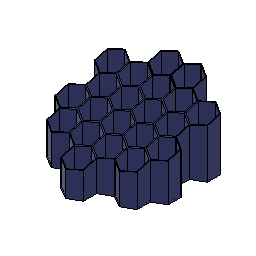
hexagon-06 (Autodesk Fusion 360 design; units mm, degrees)
Autodesk Fusion 360 part; units mm, degrees
sketch "Sketch1" plane through (0, 0, 0) normal (0, 1, 0) x (1, 0, 0)
  line L0 (15.0321, 8.6045) -> (0.0644, 17.3204)
  line L1 (0.0644, 17.3204) -> (-14.9677, 8.7159)
  line L2 (-14.9677, 8.7159) -> (-15.0321, -8.6045)
  line L3 (-15.0321, -8.6045) -> (-0.0644, -17.3204)
  line L4 (-0.0644, -17.3204) -> (14.9677, -8.7159)
  line L5 (14.9677, -8.7159) -> (15.0321, 8.6045)
  line L6 (14.9677, -8.7159) -> (-0.0644, -17.3204)
  line L7 (-0.0644, -17.3204) -> (-0.1287, -34.6408)
  line L8 (-0.1287, -34.6408) -> (14.839, -43.3567)
  line L9 (14.839, -43.3567) -> (29.8711, -34.7523)
  line L10 (29.8711, -34.7523) -> (29.9354, -17.4319)
  line L11 (29.9354, -17.4319) -> (14.9677, -8.7159)
  line L12 (14.839, -43.3567) -> (-0.1287, -34.6408)
  line L13 (-0.1287, -34.6408) -> (-15.1608, -43.2452)
  line L14 (-15.1608, -43.2452) -> (-15.2252, -60.5656)
  line L15 (-15.2252, -60.5656) -> (-0.2575, -69.2816)
  line L16 (-0.2575, -69.2816) -> (14.7746, -60.6771)
  line L17 (14.7746, -60.6771) -> (14.839, -43.3567)
  line L18 (14.2, 8.1984) -> (0, 16.3967)
  line L19 (0, 16.3967) -> (-14.2, 8.1984)
  line L20 (-14.2, 8.1984) -> (-14.2, -8.1984)
  line L21 (-14.2, -8.1984) -> (0, -16.3967)
  line L22 (0, -16.3967) -> (14.2, -8.1984)
  line L23 (14.2, -8.1984) -> (14.2, 8.1984)
  line L24 (29.1033, -17.838) -> (14.9033, -9.6396)
  line L25 (14.9033, -9.6396) -> (0.7033, -17.838)
  line L26 (0.7033, -17.838) -> (0.7033, -34.2347)
  line L27 (0.7033, -34.2347) -> (14.9033, -42.4331)
  line L28 (14.9033, -42.4331) -> (29.1033, -34.2347)
  line L29 (29.1033, -34.2347) -> (29.1033, -17.838)
  line L30 (14.0069, -43.7628) -> (-0.1931, -35.5644)
  line L31 (-0.1931, -35.5644) -> (-14.3931, -43.7628)
  line L32 (-14.3931, -43.7628) -> (-14.3931, -60.1595)
  line L33 (-14.3931, -60.1595) -> (-0.1931, -68.3579)
  line L34 (-0.1931, -68.3579) -> (14.0069, -60.1595)
  line L35 (14.0069, -60.1595) -> (14.0069, -43.7628)
  line L36 (14.7746, -60.6771) -> (-0.2575, -69.2816)
  line L37 (-0.2575, -69.2816) -> (-0.3218, -86.6019)
  line L38 (-0.3218, -86.6019) -> (14.6459, -95.3179)
  line L39 (14.6459, -95.3179) -> (29.678, -86.7134)
  line L40 (29.678, -86.7134) -> (29.7423, -69.393)
  line L41 (29.7423, -69.393) -> (14.7746, -60.6771)
  line L42 (28.9103, -69.7991) -> (14.7103, -61.6007)
  line L43 (14.7103, -61.6007) -> (0.5103, -69.7991)
  line L44 (0.5103, -69.7991) -> (0.5103, -86.1959)
  line L45 (0.5103, -86.1959) -> (14.7103, -94.3942)
  line L46 (14.7103, -94.3942) -> (28.9103, -86.1959)
  line L47 (28.9103, -86.1959) -> (28.9103, -69.7991)
  line L48 (44.7746, -60.6771) -> (29.7425, -69.2816)
  line L49 (44.9677, -8.7159) -> (45.0321, 8.6045)
  line L50 (44.9033, -9.6396) -> (30.7033, -17.838)
  line L51 (29.9356, -17.3204) -> (44.9677, -8.7159)
  line L52 (15.8, 8.1984) -> (15.8, -8.1984)
  line L53 (14.7748, -60.5656) -> (29.7425, -69.2816)
  line L54 (30, -16.3967) -> (44.2, -8.1984)
  line L55 (29.7425, -69.2816) -> (29.6782, -86.6019)
  line L56 (44.7103, -61.6007) -> (30.5103, -69.7991)
  line L57 (29.8069, -68.3579) -> (44.0069, -60.1595)
  line L58 (45.0321, 8.6045) -> (30.0644, 17.3204)
  line L59 (15.0323, 8.7159) -> (14.9679, -8.6045)
  line L60 (30.5103, -69.7991) -> (30.5103, -86.1959)
  line L61 (30.7033, -17.838) -> (30.7033, -34.2347)
  line L62 (29.8713, -34.6408) -> (14.8392, -43.2452)
  line L63 (15.8, -8.1984) -> (30, -16.3967)
  line L64 (30, 16.3967) -> (15.8, 8.1984)
  line L65 (29.8069, -35.5644) -> (15.6069, -43.7628)
  line L66 (44.839, -43.3567) -> (29.8713, -34.6408)
  line L67 (30.0644, 17.3204) -> (15.0323, 8.7159)
  line L68 (44.0069, -43.7628) -> (29.8069, -35.5644)
  line L69 (29.9356, -17.3204) -> (29.8713, -34.6408)
  line L70 (44.2, -8.1984) -> (44.2, 8.1984)
  line L71 (30.7033, -34.2347) -> (44.9033, -42.4331)
  line L72 (44.9677, -8.7159) -> (29.9356, -17.3204)
  line L73 (44.2, 8.1984) -> (30, 16.3967)
  line L74 (58.9103, -69.7991) -> (44.7103, -61.6007)
  line L75 (59.9354, -17.4319) -> (44.9677, -8.7159)
  line L76 (59.7423, -69.393) -> (44.7746, -60.6771)
  line L77 (44.9033, -42.4331) -> (59.1033, -34.2347)
  line L78 (59.678, -86.7134) -> (59.7423, -69.393)
  line L79 (59.1033, -17.838) -> (44.9033, -9.6396)
  line L80 (44.6459, -95.3179) -> (59.678, -86.7134)
  line L81 (44.839, -43.3567) -> (59.8711, -34.7523)
  line L82 (59.8711, -34.7523) -> (59.9354, -17.4319)
  line L83 (59.1033, -34.2347) -> (59.1033, -17.838)
  line L84 (15.6069, -60.1595) -> (29.8069, -68.3579)
  line L85 (44.0069, -60.1595) -> (44.0069, -43.7628)
  line L86 (29.6782, -86.6019) -> (44.6459, -95.3179)
  line L87 (30.5103, -86.1959) -> (44.7103, -94.3942)
  line L88 (14.9679, -8.6045) -> (29.9356, -17.3204)
  line L89 (29.7425, -69.2816) -> (44.7746, -60.6771)
  line L90 (29.8713, -34.6408) -> (44.839, -43.3567)
  line L91 (58.9103, -86.1959) -> (58.9103, -69.7991)
  line L92 (44.7103, -94.3942) -> (58.9103, -86.1959)
  line L93 (44.7746, -60.6771) -> (44.839, -43.3567)
  line L94 (14.8392, -43.2452) -> (14.7748, -60.5656)
  line L95 (15.6069, -43.7628) -> (15.6069, -60.1595)
  line L96 (74.7746, -60.6771) -> (59.7425, -69.2816)
  line L97 (74.9677, -8.7159) -> (75.0321, 8.6045)
  line L98 (74.9033, -9.6396) -> (60.7033, -17.838)
  line L99 (59.9356, -17.3204) -> (74.9677, -8.7159)
  line L100 (45.8, 8.1984) -> (45.8, -8.1984)
  line L101 (44.7748, -60.5656) -> (59.7425, -69.2816)
  line L102 (60, -16.3967) -> (74.2, -8.1984)
  line L103 (59.7425, -69.2816) -> (59.6782, -86.6019)
  line L104 (74.7103, -61.6007) -> (60.5103, -69.7991)
  line L105 (59.8069, -68.3579) -> (74.0069, -60.1595)
  line L106 (75.0321, 8.6045) -> (60.0644, 17.3204)
  line L107 (45.0323, 8.7159) -> (44.9679, -8.6045)
  line L108 (60.5103, -69.7991) -> (60.5103, -86.1959)
  line L109 (60.7033, -17.838) -> (60.7033, -34.2347)
  line L110 (59.8713, -34.6408) -> (44.8392, -43.2452)
  line L111 (45.8, -8.1984) -> (60, -16.3967)
  line L112 (60, 16.3967) -> (45.8, 8.1984)
  line L113 (59.8069, -35.5644) -> (45.6069, -43.7628)
  line L114 (74.839, -43.3567) -> (59.8713, -34.6408)
  line L115 (60.0644, 17.3204) -> (45.0323, 8.7159)
  line L116 (74.0069, -43.7628) -> (59.8069, -35.5644)
  line L117 (59.9356, -17.3204) -> (59.8713, -34.6408)
  line L118 (74.2, -8.1984) -> (74.2, 8.1984)
  line L119 (60.7033, -34.2347) -> (74.9033, -42.4331)
  line L120 (74.9677, -8.7159) -> (59.9356, -17.3204)
  line L121 (74.2, 8.1984) -> (60, 16.3967)
  line L122 (88.9103, -69.7991) -> (74.7103, -61.6007)
  line L123 (89.9354, -17.4319) -> (74.9677, -8.7159)
  line L124 (89.7423, -69.393) -> (74.7746, -60.6771)
  line L125 (74.9033, -42.4331) -> (89.1033, -34.2347)
  line L126 (89.678, -86.7134) -> (89.7423, -69.393)
  line L127 (89.1033, -17.838) -> (74.9033, -9.6396)
  line L128 (74.6459, -95.3179) -> (89.678, -86.7134)
  line L129 (74.839, -43.3567) -> (89.8711, -34.7523)
  line L130 (89.8711, -34.7523) -> (89.9354, -17.4319)
  line L131 (89.1033, -34.2347) -> (89.1033, -17.838)
  line L132 (45.6069, -60.1595) -> (59.8069, -68.3579)
  line L133 (74.0069, -60.1595) -> (74.0069, -43.7628)
  line L134 (59.6782, -86.6019) -> (74.6459, -95.3179)
  line L135 (60.5103, -86.1959) -> (74.7103, -94.3942)
  line L136 (44.9679, -8.6045) -> (59.9356, -17.3204)
  line L137 (59.7425, -69.2816) -> (74.7746, -60.6771)
  line L138 (59.8713, -34.6408) -> (74.839, -43.3567)
  line L139 (88.9103, -86.1959) -> (88.9103, -69.7991)
  line L140 (74.7103, -94.3942) -> (88.9103, -86.1959)
  line L141 (74.7746, -60.6771) -> (74.839, -43.3567)
  line L142 (44.8392, -43.2452) -> (44.7748, -60.5656)
  line L143 (45.6069, -43.7628) -> (45.6069, -60.1595)
  line L144 (104.7746, -60.6771) -> (89.7425, -69.2816)
  line L145 (104.9677, -8.7159) -> (105.0321, 8.6045)
  line L146 (104.9033, -9.6396) -> (90.7033, -17.838)
  line L147 (89.9356, -17.3204) -> (104.9677, -8.7159)
  line L148 (75.8, 8.1984) -> (75.8, -8.1984)
  line L149 (74.7748, -60.5656) -> (89.7425, -69.2816)
  line L150 (90, -16.3967) -> (104.2, -8.1984)
  line L151 (89.7425, -69.2816) -> (89.6782, -86.6019)
  line L152 (104.7103, -61.6007) -> (90.5103, -69.7991)
  line L153 (89.8069, -68.3579) -> (104.0069, -60.1595)
  line L154 (105.0321, 8.6045) -> (90.0644, 17.3204)
  line L155 (75.0323, 8.7159) -> (74.9679, -8.6045)
  line L156 (90.5103, -69.7991) -> (90.5103, -86.1959)
  line L157 (90.7033, -17.838) -> (90.7033, -34.2347)
  line L158 (89.8713, -34.6408) -> (74.8392, -43.2452)
  line L159 (75.8, -8.1984) -> (90, -16.3967)
  line L160 (90, 16.3967) -> (75.8, 8.1984)
  line L161 (89.8069, -35.5644) -> (75.6069, -43.7628)
  line L162 (104.839, -43.3567) -> (89.8713, -34.6408)
  line L163 (90.0644, 17.3204) -> (75.0323, 8.7159)
  line L164 (104.0069, -43.7628) -> (89.8069, -35.5644)
  line L165 (89.9356, -17.3204) -> (89.8713, -34.6408)
  line L166 (104.2, -8.1984) -> (104.2, 8.1984)
  line L167 (90.7033, -34.2347) -> (104.9033, -42.4331)
  line L168 (104.9677, -8.7159) -> (89.9356, -17.3204)
  line L169 (104.2, 8.1984) -> (90, 16.3967)
  line L170 (118.9103, -69.7991) -> (104.7103, -61.6007)
  line L171 (119.9354, -17.4319) -> (104.9677, -8.7159)
  line L172 (119.7423, -69.393) -> (104.7746, -60.6771)
  line L173 (104.9033, -42.4331) -> (119.1033, -34.2347)
  line L174 (119.678, -86.7134) -> (119.7423, -69.393)
  line L175 (119.1033, -17.838) -> (104.9033, -9.6396)
  line L176 (104.6459, -95.3179) -> (119.678, -86.7134)
  line L177 (104.839, -43.3567) -> (119.8711, -34.7523)
  line L178 (119.8711, -34.7523) -> (119.9354, -17.4319)
  line L179 (119.1033, -34.2347) -> (119.1033, -17.838)
  line L180 (75.6069, -60.1595) -> (89.8069, -68.3579)
  line L181 (104.0069, -60.1595) -> (104.0069, -43.7628)
  line L182 (89.6782, -86.6019) -> (104.6459, -95.3179)
  line L183 (90.5103, -86.1959) -> (104.7103, -94.3942)
  line L184 (74.9679, -8.6045) -> (89.9356, -17.3204)
  line L185 (89.7425, -69.2816) -> (104.7746, -60.6771)
  line L186 (89.8713, -34.6408) -> (104.839, -43.3567)
  line L187 (118.9103, -86.1959) -> (118.9103, -69.7991)
  line L188 (104.7103, -94.3942) -> (118.9103, -86.1959)
  line L189 (104.7746, -60.6771) -> (104.839, -43.3567)
  line L190 (74.8392, -43.2452) -> (74.7748, -60.5656)
  line L191 (75.6069, -43.7628) -> (75.6069, -60.1595)
  line L192 (30.0644, 17.3204) -> (45.0323, 8.7159)
  line L193 (45.0323, 8.7159) -> (59.9679, 17.3763)
  line L194 (59.9679, 17.3763) -> (59.9356, 34.6411)
  line L195 (59.9356, 34.6411) -> (44.9677, 43.2456)
  line L196 (44.9677, 43.2456) -> (30.0321, 34.5852)
  line L197 (30.0321, 34.5852) -> (30.0644, 17.3204)
  line L198 (59.9679, 17.3763) -> (75.0323, 8.7159)
  line L199 (75.0323, 8.7159) -> (90.0646, 17.4319)
  line L200 (90.0646, 17.4319) -> (90.0325, 34.8082)
  line L201 (90.0325, 34.8082) -> (74.9681, 43.4686)
  line L202 (74.9681, 43.4686) -> (59.9358, 34.7526)
  line L203 (59.9358, 34.7526) -> (59.9679, 17.3763)
  line L204 (104.9677, -8.7159) -> (119.9354, -17.4319)
  line L205 (119.9354, -17.4319) -> (134.9675, -8.8274)
  line L206 (134.9675, -8.8274) -> (135.0319, 8.493)
  line L207 (135.0319, 8.493) -> (120.0642, 17.2089)
  line L208 (120.0642, 17.2089) -> (105.0321, 8.6045)
  line L209 (105.0321, 8.6045) -> (104.9677, -8.7159)
  line L210 (104.839, -43.3567) -> (104.7746, -60.6771)
  line L211 (104.7746, -60.6771) -> (119.7423, -69.393)
  line L212 (119.7423, -69.393) -> (134.7744, -60.7886)
  line L213 (134.7744, -60.7886) -> (134.8388, -43.4682)
  line L214 (134.8388, -43.4682) -> (119.8711, -34.7523)
  line L215 (119.8711, -34.7523) -> (104.839, -43.3567)
  line L216 (44.6459, -95.3179) -> (44.678, -112.6942)
  line L217 (44.678, -112.6942) -> (59.7423, -121.3546)
  line L218 (59.7423, -121.3546) -> (74.7746, -112.6386)
  line L219 (74.7746, -112.6386) -> (74.7425, -95.2623)
  line L220 (74.7425, -95.2623) -> (59.6782, -86.6019)
  line L221 (59.6782, -86.6019) -> (44.6459, -95.3179)
  line L222 (59.2161, 34.1512) -> (45.0323, 42.3775)
  line L223 (45.0323, 42.3775) -> (30.8162, 34.2071)
  line L224 (30.8162, 34.2071) -> (30.7839, 17.8104)
  line L225 (30.7839, 17.8104) -> (44.9677, 9.584)
  line L226 (44.9677, 9.584) -> (59.1838, 17.7544)
  line L227 (59.1838, 17.7544) -> (59.2161, 34.1512)
  line L228 (89.2002, 34.2906) -> (75.0002, 42.489)
  line L229 (75.0002, 42.489) -> (60.8002, 34.2906)
  line L230 (60.8002, 34.2906) -> (60.8002, 17.8939)
  line L231 (60.8002, 17.8939) -> (75.0002, 9.6955)
  line L232 (75.0002, 9.6955) -> (89.2002, 17.8939)
  line L233 (89.2002, 17.8939) -> (89.2002, 34.2906)
  line L234 (134.0371, -43.9271) -> (119.8676, -35.676)
  line L235 (119.8676, -35.676) -> (105.6373, -43.8216)
  line L236 (105.6373, -43.8216) -> (105.5763, -60.2182)
  line L237 (105.5763, -60.2182) -> (119.7458, -68.4693)
  line L238 (119.7458, -68.4693) -> (133.9761, -60.3237)
  line L239 (133.9761, -60.3237) -> (134.0371, -43.9271)
  line L240 (134.2302, 8.0341) -> (120.0607, 16.2852)
  line L241 (120.0607, 16.2852) -> (105.8304, 8.1396)
  line L242 (105.8304, 8.1396) -> (105.7694, -8.257)
  line L243 (105.7694, -8.257) -> (119.9389, -16.5081)
  line L244 (119.9389, -16.5081) -> (134.1692, -8.3626)
  line L245 (134.1692, -8.3626) -> (134.2302, 8.0341)
  line L246 (73.8951, -95.7537) -> (59.68, -87.5815)
  line L247 (59.68, -87.5815) -> (45.4951, -95.8061)
  line L248 (45.4951, -95.8061) -> (45.5254, -112.2028)
  line L249 (45.5254, -112.2028) -> (59.7405, -120.375)
  line L250 (59.7405, -120.375) -> (73.9254, -112.1504)
  line L251 (73.9254, -112.1504) -> (73.8951, -95.7537)
  point P0 (14.9033, -26.0363)
  point P1 (-0.1931, -51.9612)
  point P2 (14.9033, -26.0363)
  point P3 (-0.1931, -51.9612)
  point P4 (14.7103, -77.9975)
  point P5 (14.7103, -77.9975)
  point P6 (44.9033, -26.0363)
  point P7 (29.8069, -51.9612)
  point P8 (44.9033, -26.0363)
  point P9 (30, 0)
  point P10 (30, 0)
  point P11 (29.8069, -51.9612)
  point P12 (44.7103, -77.9975)
  point P13 (30, 0)
  point P14 (44.7103, -77.9975)
  point P15 (74.9033, -26.0363)
  point P16 (59.8069, -51.9612)
  point P17 (74.9033, -26.0363)
  point P18 (60, 0)
  point P19 (60, 0)
  point P20 (59.8069, -51.9612)
  point P21 (74.7103, -77.9975)
  point P22 (60, 0)
  point P23 (74.7103, -77.9975)
  point P24 (104.9033, -26.0363)
  point P25 (89.8069, -51.9612)
  point P26 (104.9033, -26.0363)
  point P27 (90, 0)
  point P28 (90, 0)
  point P29 (89.8069, -51.9612)
  point P30 (104.7103, -77.9975)
  point P31 (90, 0)
  point P32 (104.7103, -77.9975)
  point P33 (59.8713, -34.6408)
  point P34 (45, 25.9808)
  point P35 (75.0002, 26.0922)
  point P36 (119.9998, -0.1115)
  point P37 (119.8067, -52.0726)
  point P38 (59.7103, -103.9783)
  point P39 (45, 25.9808)
  point P40 (75.0002, 26.0922)
  point P41 (119.8067, -52.0726)
  point P42 (119.9998, -0.1115)
  point P43 (59.7103, -103.9783)
  dimension "d29" = 15
  dimension "d30" = 14.2
  dimension "d31" = 14.2
  dimension "d32" = 14.2
  dimension "d33" = 14.2
  dimension "d36" = 90
  dimension "d37" = 0
  dimension "d47" = 14.2
  dimension "d48" = 14.2
  dimension "d49" = 14.2
  dimension "d50" = 14.2
  dimension "d51" = 14.2
  constraint coincident P2 P0
  constraint coincident P3 P1
  constraint coincident P5 P4
  constraint coincident P33 L110.start
  constraint coincident P39 P34
  constraint coincident P40 P35
  constraint coincident P41 P37
  constraint coincident P42 P36
  constraint coincident P43 P38
  measures "d29" distance of origin L5
  measures "d30" distance of origin L23
  measures "d31" distance of P2 L29
  measures "d32" distance of P3 L35
  measures "d33" distance of P5 L47
  measures "d47" distance of P39 L227
  measures "d48" distance of P40 L233
  measures "d49" distance of P41 L239
  measures "d50" distance of P42 L245
  measures "d51" distance of P43 L251
extrude "Extrude2" add sketch "Sketch1" along normal blind 1.6 contours L0 L5 L59 L88 | L0 L5 L49 L51 L58 L59 L67 L72 L88 L107 L136 | L0 L1 L2 L3 L4 L5 L6 L59 L88 | L5 L11 L69 L88 | L4 L6 L7 L8 L11 L12 L62 L69 L94 | L10 L11 L51 L66 L69 L72 L75 L90 L110 L117 L142 | L192 L193 L194 L195 L196 L197 | L10 L11 L66 L69 L90 | L49 L75 L117 L136 | L49 L58 L97 L99 L106 L107 L115 L120 L136 L155 L184 | L49 L58 L107 L136 | L8 L12 L13 L14 L15 L16 L17 L36 L53 L94 | L8 L9 L10 L12 L62 L66 L90 L94 | L75 L82 L99 L114 L117 L120 L123 L138 L158 L165 L190 | L75 L82 L114 L117 L138 | L198 L199 L200 L201 L202 L203 | L8 L12 L17 L53 L94 | L9 L10 L17 L48 L53 L66 L89 L90 L93 L101 L142 | L66 L81 L82 L90 L110 L114 L138 L142 | L97 L106 L145 L147 L154 L155 L163 L168 L184 L209 | L97 L106 L155 L184 | L66 L90 L93 L101 L142 | L97 L123 L165 L184 | L81 L82 L93 L96 L101 L114 L137 L138 L141 L149 L190 | L17 L41 L53 L55 | L16 L36 L37 L38 L39 L40 L41 L55 L86 | L123 L130 L147 L162 L165 L168 L171 L177 L178 L186 L204 L215 | L123 L130 L162 L165 L186 | L114 L129 L130 L138 L158 L162 L186 L190 | L114 L138 L141 L149 L190 | L145 L171 L204 L205 L206 L207 L208 L209 | L40 L41 L48 L55 L76 L86 L89 L103 L221 | L76 L93 L101 L103 | L129 L130 L141 L144 L149 L162 L185 L186 L189 L210 | L40 L41 L55 L86 | L76 L78 L96 L103 L124 L126 L128 L137 L151 L182 L219 L220 | L124 L141 L149 L151 | L76 L78 L103 L134 L220 | L172 L177 L189 L210 L211 L212 L213 L214 L215 | L124 L126 L144 L151 L172 L174 L176 L182 L185 L211 | L78 L80 L134 L220 L221 | L124 L126 L151 L182 | L78 L80 L128 L134 L216 L217 L218 L219 | L128 L134 L219 L220 | L18 L19 L20 L21 L22 L23 | L24 L25 L26 L27 L28 L29 | L30 L31 L32 L33 L34 L35 | L42 L43 L44 L45 L46 L47 | L50 L61 L71 L77 L79 L83 | L52 L54 L63 L64 L70 L73 | L56 L60 L74 L87 L91 L92 | L57 L65 L68 L84 L85 L95 | L98 L109 L119 L125 L127 L131 | L100 L102 L111 L112 L118 L121 | L104 L108 L122 L135 L139 L140 | L105 L113 L116 L132 L133 L143 | L146 L157 L167 L173 L175 L179 | L148 L150 L159 L160 L166 L169 | L152 L156 L170 L183 L187 L188 | L153 L161 L164 L180 L181 L191 | L222 L223 L224 L225 L226 L227 | L228 L229 L230 L231 L232 L233 | L234 L235 L236 L237 L238 L239 | L240 L241 L242 L243 L244 L245 | L246 L247 L248 L249 L250 L251 makes body 1
extrude "Extrude3" add sketch "Sketch1" along normal blind 80 contours L0 L5 L59 L88 | L0 L5 L49 L51 L58 L59 L67 L72 L88 L107 L136 | L0 L1 L2 L3 L4 L5 L6 L59 L88 | L5 L11 L69 L88 | L4 L6 L7 L8 L11 L12 L62 L69 L94 | L10 L11 L51 L66 L69 L72 L75 L90 L110 L117 L142 | L192 L193 L194 L195 L196 L197 | L10 L11 L66 L69 L90 | L49 L75 L117 L136 | L49 L58 L97 L99 L106 L107 L115 L120 L136 L155 L184 | L49 L58 L107 L136 | L8 L12 L13 L14 L15 L16 L17 L36 L53 L94 | L8 L9 L10 L12 L62 L66 L90 L94 | L75 L82 L99 L114 L117 L120 L123 L138 L158 L165 L190 | L75 L82 L114 L117 L138 | L198 L199 L200 L201 L202 L203 | L8 L12 L17 L53 L94 | L9 L10 L17 L48 L53 L66 L89 L90 L93 L101 L142 | L66 L81 L82 L90 L110 L114 L138 L142 | L97 L106 L145 L147 L154 L155 L163 L168 L184 L209 | L97 L106 L155 L184 | L66 L90 L93 L101 L142 | L97 L123 L165 L184 | L81 L82 L93 L96 L101 L114 L137 L138 L141 L149 L190 | L17 L41 L53 L55 | L16 L36 L37 L38 L39 L40 L41 L55 L86 | L123 L130 L147 L162 L165 L168 L171 L177 L178 L186 L204 L215 | L123 L130 L162 L165 L186 | L114 L129 L130 L138 L158 L162 L186 L190 | L114 L138 L141 L149 L190 | L145 L171 L204 L205 L206 L207 L208 L209 | L40 L41 L48 L55 L76 L86 L89 L103 L221 | L76 L93 L101 L103 | L129 L130 L141 L144 L149 L162 L185 L186 L189 L210 | L40 L41 L55 L86 | L76 L78 L96 L103 L124 L126 L128 L137 L151 L182 L219 L220 | L124 L141 L149 L151 | L76 L78 L103 L134 L220 | L172 L177 L189 L210 L211 L212 L213 L214 L215 | L124 L126 L144 L151 L172 L174 L176 L182 L185 L211 | L78 L80 L134 L220 L221 | L124 L126 L151 L182 | L78 L80 L128 L134 L216 L217 L218 L219 | L128 L134 L219 L220 bodies 1
sketch "Sketch2" plane through (0, 0, 0) normal (1, 0, 0) x (0, 0, -1)
  line L0 (58.2994, 83.577) -> (-124.7141, 32.2408)
  line L1 (-124.7141, 32.2408) -> (-124.7141, 83.577)
  line L2 (-124.7141, 83.577) -> (58.2994, 83.577)
  constraint vertical L1
  constraint perpendicular L1 L2
extrude "Extrude4" cut sketch "Sketch2" along normal blind 159 and the other way blind 41 bodies 1
copy_body "Body->Comp1" bodies 1 removing the originals makes body 2 in component "hexagon-06"
component "hexagon-06" placed x (1, 0, 0) y (0, 1, 0) z (0, 0, 1) at (0, 0, 0)
equation "size1 = 15 mm"
equation "offset1 = 0.8 mm"
equation "d29 = size1"
equation "d30 = size1 - offset1"
equation "d31 = size1 - offset1"
equation "d32 = size1 - offset1"
equation "d33 = size1 - offset1"
equation "d36 = 6 * size1"
equation "d38 = 2 * offset1"
equation "d40 = height"
equation "height = 80 mm"
equation "d47 = size1 - offset1"
equation "d48 = size1 - offset1"
equation "d49 = size1 - offset1"
equation "d50 = size1 - offset1"
equation "d51 = size1 - offset1"
